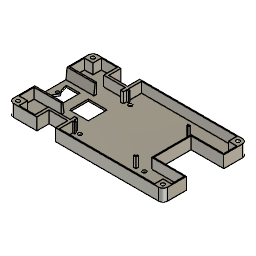
CAR (Autodesk Fusion 360 archive; units mm, degrees)
design "MID"
Autodesk Fusion 360 part; units mm, degrees
(part 1 of 2)
sketch "Sketch1" plane through (0, 0, 0) normal (0, 0, 1) x (1, 0, 0)
  line L0 (0, 0) -> (165, 0)
  line L1 (165, 0) -> (165, 90)
  line L2 (165, 90) -> (0, 90)
  line L3 (0, 90) -> (0, 0)
  dimension "d1" = 165
  dimension "d2" = 90
  constraint horizontal L0
  constraint vertical L1
  constraint horizontal L2
  constraint vertical L3
  constraint coincident L0.start L3.end
  measures "d1" distance of L0.start L0.end
  measures "d2" distance of L0.start L2.end
extrude "Extrude1" add sketch "Sketch1" along normal blind 3
sketch "Sketch4" plane through (0, 0, 3) normal (0, 0, 1) x (-1, 0, 0)
  line L0 (-165, 0) -> (-165, -90)
  line L1 (-165, -90) -> (0, -90)
  line L2 (0, -90) -> (0, 0)
  line L3 (0, 0) -> (-165, 0)
  line L4 (-30, -90) -> (-50, -90)
  line L5 (-50, -90) -> (-50, -77)
  line L6 (-50, -77) -> (-30, -77)
  line L7 (-30, -77) -> (-30, -90)
  line L8 (-30, 0) -> (-50, 0)
  line L9 (-50, 0) -> (-50, -13)
  line L10 (-50, -13) -> (-30, -13)
  line L11 (-30, -13) -> (-30, 0)
  dimension "d9" = 20
  dimension "d10" = 13
  dimension "d11" = 20
  dimension "d12" = 13
  constraint horizontal L4
  constraint vertical L5
  constraint horizontal L6
  constraint vertical L7
  constraint coincident L1 L4.start
  constraint horizontal L8
  constraint vertical L9
  constraint horizontal L10
  constraint vertical L11
  constraint coincident L3 L8.start
  measures "d9" distance of L4.start L4.end
  measures "d10" distance of L4.start L6.end
  measures "d11" distance of L8.start L8.end
  measures "d12" distance of L8.start L10.end
extrude "Extrude2" cut sketch "Sketch4" against normal blind 3 contours L3 L8 L9 L10 L11 | L1 L4 L5 L6 L7
sketch "Sketch6" plane through (0, 0, 3) normal (0, 0, 1) x (-1, 0, 0)
  line L0 (-30, -77) -> (-30, -90)
  line L1 (-30, -90) -> (0, -90)
  line L2 (0, -90) -> (0, 0)
  line L3 (0, 0) -> (-30, 0)
  line L4 (-30, 0) -> (-30, -13)
  line L5 (-30, -13) -> (-50, -13)
  line L6 (-50, -13) -> (-50, 0)
  line L7 (-50, 0) -> (-165, 0)
  line L8 (-165, 0) -> (-165, -90)
  line L9 (-50, -90) -> (-50, -77)
  line L10 (-50, -77) -> (-30, -77)
  line L11 (-5, -45) -> (-5, -60)
  line L12 (-5, -60) -> (-20, -60)
  line L13 (-20, -60) -> (-20, -30)
  line L14 (-20, -30) -> (-5, -30)
  line L15 (-5, -30) -> (-5, -45)
  line L16 (0, -65) -> (-25, -65)
  line L17 (-25, -65) -> (-25, -25)
  line L18 (-25, -25) -> (0, -25)
  line L19 (0, -25) -> (0, -65)
  line L20 (-165, -90) -> (-50, -90)
  dimension "d20" = 15
  dimension "d21" = 15
  constraint parallel L2 L11
  constraint perpendicular L2 L12
  constraint perpendicular L12 L13
  constraint perpendicular L2 L14
  constraint perpendicular L14 L15
  constraint horizontal L16
  constraint vertical L17
  constraint horizontal L18
  constraint vertical L19
  constraint coincident L2 L16.start
  measures "d20" distance of L11.start L11.end
  measures "d21" distance of L11.end L12.end
extrude "Extrude4" add sketch "Sketch6" along normal blind 10 contours L2 L16 L17 L18 L19
sketch "Sketch7" plane through (0, 0, 3) normal (0, 0, 1) x (-1, 0, 0)
  line L0 (0, -65) -> (-25, -65)
  line L1 (-25, -65) -> (-25, -25)
  line L2 (-25, -25) -> (0, -25)
  line L3 (0, -25) -> (0, 0)
  line L4 (0, 0) -> (-30, 0)
  line L5 (-30, 0) -> (-30, -13)
  line L6 (-30, -13) -> (-50, -13)
  line L7 (-50, -13) -> (-50, 0)
  line L8 (-50, 0) -> (-165, 0)
  line L9 (-165, 0) -> (-165, -90)
  line L10 (-165, -90) -> (-50, -90)
  line L11 (-50, -90) -> (-50, -77)
  line L12 (-50, -77) -> (-30, -77)
  line L13 (-30, -77) -> (-30, -90)
  line L14 (-30, -90) -> (0, -90)
  line L15 (-25, 0) -> (-55, 0)
  line L16 (-55, 0) -> (-55, -15)
  line L17 (-55, -15) -> (-25, -15)
  line L18 (-25, -15) -> (-25, 0)
  line L19 (-25, -90) -> (-55, -90)
  line L20 (-55, -90) -> (-55, -75)
  line L21 (-55, -75) -> (-25, -75)
  line L22 (-25, -75) -> (-25, -90)
  line L23 (0, -90) -> (0, -65)
  constraint horizontal L15
  constraint vertical L16
  constraint horizontal L17
  constraint vertical L18
  constraint coincident L4 L15.start
  constraint horizontal L19
  constraint vertical L20
  constraint horizontal L21
  constraint vertical L22
  constraint coincident L14 L19.start
extrude "Extrude5" add sketch "Sketch7" along normal blind 10 contours L10 L11 L12 L13 L14 L19 L20 L21 L22 | L4 L5 L6 L7 L8 L15 L16 L17 L18
sketch "Sketch12" plane through (0, 0, 3) normal (0, 0, 1) x (-1, 0, 0)
  line L0 (-55, -15) -> (-55, 0)
  line L1 (-55, 0) -> (-165, 0)
  line L2 (-165, 0) -> (-165, -90)
  line L3 (-165, -90) -> (-55, -90)
  line L4 (-55, -90) -> (-55, -75)
  line L5 (-55, -75) -> (-25, -75)
  line L6 (-25, -75) -> (-25, -90)
  line L7 (-25, -90) -> (0, -90)
  line L8 (0, -90) -> (0, -65)
  line L9 (0, -65) -> (-25, -65)
  line L10 (-25, -65) -> (-25, -25)
  line L11 (-25, -25) -> (0, -25)
  line L12 (0, -25) -> (0, 0)
  line L13 (0, 0) -> (-25, 0)
  line L14 (-25, 0) -> (-25, -15)
  line L15 (-25, -15) -> (-55, -15)
  line L16 (-25, -90) -> (0, -90)
  line L17 (0, -90) -> (0, -65)
  line L18 (0, -65) -> (-5, -65)
  line L19 (-5, -65) -> (-5, -85)
  line L20 (-5, -85) -> (-25, -85)
  line L21 (-25, -85) -> (-25, -90)
  line L22 (0, -25) -> (0, 0)
  line L23 (0, 0) -> (-25, 0)
  line L24 (-25, 0) -> (-25, -5)
  line L25 (-25, -5) -> (-5, -5)
  line L26 (-5, -5) -> (-5, -25)
  line L27 (-5, -25) -> (0, -25)
  line L28 (-55, -90) -> (-165, -90)
  line L29 (-165, -90) -> (-165, 0)
  line L30 (-165, 0) -> (-55, 0)
  line L31 (-55, 0) -> (-55, -5)
  line L32 (-55, -5) -> (-160, -5)
  line L33 (-160, -5) -> (-160, -85)
  line L34 (-160, -85) -> (-55, -85)
  line L35 (-55, -90) -> (-55, -85)
  constraint coincident L6.end L7.start
  constraint coincident L7.end L8.start
  constraint coincident L8.end L9.start
  constraint coincident L9 L18.end
  constraint perpendicular L18 L19
  constraint coincident L6 L20.end
  constraint perpendicular L6 L20
  constraint coincident L11.end L12.start
  constraint coincident L12.end L13.start
  constraint coincident L13.end L14.start
  constraint coincident L14 L24.end
  constraint perpendicular L24 L25
  constraint coincident L11 L26.end
  constraint perpendicular L11 L26
  constraint coincident L3.end L4.start
  constraint coincident L2.end L3.start
  constraint coincident L1.end L2.start
  constraint coincident L0.end L1.start
  constraint coincident L0 L31.end
  constraint perpendicular L31 L32
  constraint perpendicular L32 L33
  constraint coincident L4 L34.end
  constraint perpendicular L4 L34
extrude "Extrude9" add sketch "Sketch12" along normal blind 10 contours L0 L1 L2 L3 L4 L28 L29 L30 L31 L32 L33 L34 L35 | L11 L12 L13 L14 L22 L23 L24 L25 L26 L27 | L6 L7 L8 L9 L16 L17 L18 L19 L20 L21
fillet "Fillet6" radius 5 4 edges at (0, 0, 6.5) (165, 0, 6.5) (165, 90, 6.5) (0, 90, 6.5)
extrude "Extrude10" add 1 faces at (45, 75, 6.3333) along direction (0, -1, 0) blind 2.5
extrude "Extrude11" add 1 faces at (45, 15, 6.3333) along direction (0, 1, 0) blind 2.5
extrude "Extrude12" cut 1 faces at (10, 40, 3) along direction (0, 0, -1) blind 3
sketch "Sketch13" plane through (0, 0, 3) normal (0, 0, 1) x (-1, 0, 0)
  line L0 (-55, -17.5) -> (-55, -5)
  line L1 (-55, -5) -> (-160, -5)
  line L2 (-160, -5) -> (-160, -85)
  line L3 (-160, -85) -> (-55, -85)
  line L4 (-55, -85) -> (-55, -72.5)
  line L5 (-55, -72.5) -> (-25, -72.5)
  line L6 (-25, -72.5) -> (-25, -85)
  line L7 (-25, -85) -> (-5, -85)
  line L8 (-5, -85) -> (-5, -65)
  line L9 (-5, -65) -> (-25, -65)
  line L10 (-25, -65) -> (-25, -25)
  line L11 (-25, -25) -> (-5, -25)
  line L12 (-5, -25) -> (-5, -5)
  line L13 (-5, -5) -> (-25, -5)
  line L14 (-25, -5) -> (-25, -17.5)
  line L15 (-25, -17.5) -> (-55, -17.5)
  line L16 (-30, -55) -> (-50, -55)
  line L17 (-50, -55) -> (-50, -35)
  line L18 (-50, -35) -> (-30, -35)
  line L19 (-30, -35) -> (-30, -55)
  constraint horizontal L16
  constraint vertical L17
  constraint horizontal L18
  constraint vertical L19
extrude "Extrude13" cut sketch "Sketch13" against normal blind 3 contours L16 L17 L18 L19
sketch "Sketch15" plane through (0, 0, 3) normal (0, 0, 1) x (-1, 0, 0)
  line L0 (-50, -55) -> (-50, -35)
  line L1 (-50, -35) -> (-30, -35)
  line L2 (-30, -35) -> (-30, -55)
  line L3 (-30, -55) -> (-50, -55)
  line L4 (-55, -17.5) -> (-55, -5)
  line L5 (-55, -5) -> (-160, -5)
  line L6 (-160, -5) -> (-160, -85)
  line L7 (-160, -85) -> (-55, -85)
  line L8 (-55, -85) -> (-55, -72.5)
  line L9 (-55, -72.5) -> (-25, -72.5)
  line L10 (-25, -72.5) -> (-25, -85)
  line L11 (-25, -85) -> (-5, -85)
  line L12 (-5, -85) -> (-5, -65)
  line L13 (-5, -65) -> (-25, -65)
  line L14 (-25, -65) -> (-25, -25)
  line L15 (-25, -25) -> (-5, -25)
  line L16 (-5, -25) -> (-5, -5)
  line L17 (-5, -5) -> (-25, -5)
  line L18 (-25, -5) -> (-25, -17.5)
  line L19 (-25, -17.5) -> (-55, -17.5)
  line L20 (-5, -85) -> (-10, -85)
  line L21 (-10, -85) -> (-10, -80)
  line L22 (-10, -80) -> (-5, -80)
  line L23 (-5, -80) -> (-5, -85)
  line L24 (-5, -10) -> (-10, -10)
  line L25 (-10, -10) -> (-10, -5)
  line L26 (-10, -5) -> (-5, -5)
  line L27 (-5, -5) -> (-5, -10)
  line L28 (-155, -85) -> (-160, -85)
  line L29 (-160, -85) -> (-160, -80)
  line L30 (-160, -80) -> (-155, -80)
  line L31 (-155, -80) -> (-155, -85)
  line L32 (-155, -10) -> (-160, -10)
  line L33 (-160, -10) -> (-160, -5)
  line L34 (-160, -5) -> (-155, -5)
  line L35 (-155, -5) -> (-155, -10)
  constraint horizontal L20
  constraint vertical L21
  constraint horizontal L22
  constraint vertical L23
  constraint coincident L11.end L12.start
  constraint horizontal L24
  constraint vertical L25
  constraint horizontal L26
  constraint vertical L27
  constraint coincident L17 L25.end
  constraint coincident L16 L24.start
  constraint horizontal L28
  constraint vertical L29
  constraint horizontal L30
  constraint vertical L31
  constraint coincident L6 L29.end
  constraint coincident L7 L28.start
  constraint horizontal L32
  constraint vertical L33
  constraint horizontal L34
  constraint vertical L35
  constraint coincident L6 L5.end
extrude "Extrude14" add sketch "Sketch15" along normal blind 10 contours L5 L6 L32 L33 L34 L35 | L16 L17 L24 L25 L26 L27 | L6 L7 L28 L29 L30 L31 | L11 L12 L20 L21 L22 L23
sketch "Sketch16" plane through (0, 0, 13) normal (0, 0, 1) x (-1, 0, 0)
  line L0 (-55, -5) -> (-55, -17.5)
  line L1 (-55, -17.5) -> (-25, -17.5)
  line L2 (-25, -17.5) -> (-25, -5)
  line L3 (-25, -5) -> (-10, -5)
  line L4 (-10, -5) -> (-10, -10)
  line L5 (-10, -10) -> (-5, -10)
  line L6 (-5, -10) -> (-5, -25)
  line L7 (-5, -25) -> (-25, -25)
  line L8 (-25, -25) -> (-25, -65)
  line L9 (-25, -65) -> (-5, -65)
  line L10 (-5, -65) -> (-5, -80)
  line L11 (-5, -80) -> (-10, -80)
  line L12 (-10, -80) -> (-10, -85)
  line L13 (-10, -85) -> (-25, -85)
  line L14 (-25, -85) -> (-25, -72.5)
  line L15 (-25, -72.5) -> (-55, -72.5)
  line L16 (-55, -72.5) -> (-55, -85)
  line L17 (-55, -85) -> (-155, -85)
  line L18 (-155, -85) -> (-155, -80)
  line L19 (-155, -80) -> (-160, -80)
  line L20 (-160, -80) -> (-160, -10)
  line L21 (-160, -10) -> (-155, -10)
  line L22 (-155, -10) -> (-155, -5)
  line L23 (-155, -5) -> (-55, -5)
  line L24 (-20, -30) -> (-5, -30)
  line L25 (-5, -30) -> (-5, -60)
  line L26 (-5, -60) -> (-20, -60)
  line L27 (-20, -60) -> (-20, -30)
  arc A0 (-5, -90) -> (0, -85) centre (-5, -85) ccw
  line L28 (0, -85) -> (0, -5)
  arc A1 (0, -5) -> (-5, 0) centre (-5, -5) ccw
  line L29 (-5, 0) -> (-30, 0)
  line L30 (-30, 0) -> (-30, -13)
  line L31 (-30, -13) -> (-50, -13)
  line L32 (-50, -13) -> (-50, 0)
  line L33 (-50, 0) -> (-160, 0)
  arc A2 (-160, 0) -> (-165, -5) centre (-160, -5) ccw
  line L34 (-165, -5) -> (-165, -85)
  arc A3 (-165, -85) -> (-160, -90) centre (-160, -85) ccw
  line L35 (-160, -90) -> (-50, -90)
  line L36 (-50, -90) -> (-50, -77)
  line L37 (-50, -77) -> (-30, -77)
  line L38 (-30, -77) -> (-30, -90)
  line L39 (-30, -90) -> (-5, -90)
  circle A4 centre (-5, -85) radius 2
  circle A5 centre (-5, -5) radius 2
  circle A6 centre (-160, -85) radius 2
  circle A7 centre (-160, -5) radius 2
  dimension "d52" = 4
  dimension "d53" = 4
  dimension "d54" = 4
  dimension "d55" = 4
  constraint concentric A0 A4
  constraint concentric A1 A5
  constraint concentric A3 A6
  constraint concentric A2 A7
  measures "d52" diameter of A4
  measures "d53" diameter of A5
  measures "d54" diameter of A6
  measures "d55" diameter of A7
extrude "Extrude15" cut sketch "Sketch16" against normal blind 13 contours A4 | A5 | A6 | A7
sketch "Sketch17" plane through (0, 0, 3) normal (0, 0, 1) x (-1, 0, 0)
  line L0 (-50, -55) -> (-50, -35)
  line L1 (-50, -35) -> (-30, -35)
  line L2 (-30, -35) -> (-30, -55)
  line L3 (-30, -55) -> (-50, -55)
  line L4 (-160, -80) -> (-155, -80)
  line L5 (-155, -80) -> (-155, -85)
  line L6 (-155, -85) -> (-55, -85)
  line L7 (-55, -85) -> (-55, -72.5)
  line L8 (-55, -72.5) -> (-25, -72.5)
  line L9 (-25, -72.5) -> (-25, -85)
  line L10 (-25, -85) -> (-10, -85)
  line L11 (-10, -85) -> (-10, -80)
  line L12 (-10, -80) -> (-5, -80)
  line L13 (-5, -80) -> (-5, -65)
  line L14 (-5, -65) -> (-25, -65)
  line L15 (-25, -65) -> (-25, -25)
  line L16 (-25, -25) -> (-5, -25)
  line L17 (-5, -25) -> (-5, -10)
  line L18 (-5, -10) -> (-10, -10)
  line L19 (-10, -10) -> (-10, -5)
  line L20 (-10, -5) -> (-25, -5)
  line L21 (-25, -5) -> (-25, -17.5)
  line L22 (-25, -17.5) -> (-55, -17.5)
  line L23 (-55, -17.5) -> (-55, -5)
  line L24 (-55, -5) -> (-155, -5)
  line L25 (-155, -5) -> (-155, -10)
  line L26 (-155, -10) -> (-160, -10)
  line L27 (-160, -10) -> (-160, -80)
  line L28 (-65, -73) -> (-129, -73)
  line L29 (-129, -73) -> (-129, -17)
  line L30 (-129, -17) -> (-65, -17)
  line L31 (-65, -17) -> (-65, -73)
  line L32 (-60, -78) -> (-134, -78)
  line L33 (-134, -78) -> (-134, -12)
  line L34 (-134, -12) -> (-60, -12)
  line L35 (-60, -12) -> (-60, -78)
  dimension "d58" = 64
  dimension "d59" = 56
  dimension "d60" = 74
  dimension "d61" = 66
  constraint horizontal L28
  constraint vertical L29
  constraint horizontal L30
  constraint vertical L31
  constraint horizontal L32
  constraint vertical L33
  constraint horizontal L34
  constraint vertical L35
  measures "d58" distance of L28.start L28.end
  measures "d59" distance of L28.start L30.end
  measures "d60" distance of L32.start L32.end
  measures "d61" distance of L32.start L34.end
extrude "Extrude18" add 1 faces at (10, 30, 8.6667) along direction (0, 1, 0) blind 4
extrude "Extrude19" add 1 faces at (15, 60, 8.6667) along direction (0, -1, 0) blind 4
extrude "Extrude20" cut 1 faces at (18.3333, 25, 6.3333) along direction (0, 1, 0) blind 4
extrude "Extrude21" cut 1 faces at (11.6667, 65, 6.3333) along direction (0, -1, 0) blind 4
sketch "Sketch19" plane through (0, 0, 0) normal (0, 0, 1) x (1, 0, 0)
  spline S0 degree 5 poles (5, 34) (5.1175, 33.9082) (5.3447, 33.8543) (5.6451, 34.1512) (5.923, 35.197) (6.2299, 37.171) (6.6925, 39.3464) (7.4607, 41.3157) (8.4564, 42.8586) (9.4177, 43.9473) (10.0442, 44.686) (10.0986, 45.2722) (9.5576, 45.9525) (8.6258, 46.9693) (7.5898, 48.4821) (6.7224, 50.5039) (6.1493, 52.81) (5.7864, 54.9179) (5.4759, 56.2775) (5.0616, 56.4098) (4.5396, 55.0911) (4.0446, 52.4587) (3.6617, 48.8489) (3.4755, 44.7456) (3.5326, 40.6932) (3.848, 37.226) (4.2676, 35.2762) (4.6394, 34.4052) (4.8825, 34.0918) (5, 34) knots 0 0 0 0 0 0 0.04 0.08 0.12 0.16 0.2 0.24 0.28 0.32 0.36 0.4 0.44 0.48 0.52 0.56 0.6 0.64 0.68 0.72 0.76 0.8 0.84 0.88 0.92 0.96 1 1 1 1 1 1
  line L0 (4.4073, 34.463) -> (5.5927, 33.537)
  line L1 (5.3989, 56.5988) -> (4.6011, 55.4012)
  point P0 (7, 40)
  point P1 (10, 45)
  point P2 (7, 50)
  point P3 (5, 56)
  constraint midpoint S0.start L0
  constraint midpoint P3 L1
extrude "Extrude22" add sketch "Sketch19" along normal blind 3
sketch "Sketch20" plane through (0, 0, 0) normal (0, 0, -1) x (1, 0, 0)
  arc A0 (0, -85) -> (5, -90) centre (5, -85) ccw
  line L0 (5, -90) -> (30, -90)
  line L1 (30, -90) -> (30, -77)
  line L2 (30, -77) -> (50, -77)
  line L3 (50, -77) -> (50, -90)
  line L4 (50, -90) -> (160, -90)
  arc A1 (160, -90) -> (165, -85) centre (160, -85) ccw
  line L5 (165, -85) -> (165, -5)
  arc A2 (165, -5) -> (160, 0) centre (160, -5) ccw
  line L6 (160, 0) -> (50, 0)
  line L7 (50, 0) -> (50, -13)
  line L8 (50, -13) -> (30, -13)
  line L9 (30, -13) -> (30, 0)
  line L10 (30, 0) -> (5, 0)
  arc A3 (5, 0) -> (0, -5) centre (5, -5) ccw
  line L11 (0, -5) -> (0, -85)
  line L12 (50, -35) -> (50, -55)
  line L13 (50, -55) -> (30, -55)
  line L14 (30, -55) -> (30, -35)
  line L15 (30, -35) -> (50, -35)
  circle A4 centre (5, -85) radius 2
  circle A5 centre (160, -85) radius 2
  circle A6 centre (5, -5) radius 2
  circle A7 centre (160, -5) radius 2
  spline S0 degree 5 poles (5.399, -34) (5.4257, -34.0237) (5.5488, -34.1551) (5.7455, -34.5509) (5.9678, -35.4853) (6.2299, -37.171) (6.6925, -39.3464) (7.4607, -41.3157) (8.4564, -42.8586) (9.4177, -43.9473) (10.0442, -44.686) (10.0986, -45.2722) (9.5576, -45.9525) (8.6258, -46.9693) (7.5898, -48.4821) (6.7224, -50.5039) (6.1493, -52.81) (5.8561, -54.5129) (5.6598, -55.4485) (5.5168, -55.8531) (5.4396, -55.9947) (5.4367, -56) knots 0.029213 0.029213 0.029213 0.029213 0.029213 0.029213 0.04 0.08 0.12 0.16 0.2 0.24 0.28 0.32 0.36 0.4 0.44 0.48 0.52 0.56 0.6 0.64 0.641569 0.641569 0.641569 0.641569 0.641569 0.641569
  line L16 (5.399, -34) -> (20, -34)
  line L17 (20, -34) -> (20, -56)
  line L18 (20, -56) -> (5.4367, -56)
  circle A8 centre (7, -45) radius 1.5
  dimension "d76" = 3
  measures "d76" diameter of A8
extrude "Extrude23" cut sketch "Sketch20" against normal blind 3 contours A8
extrude "Extrude26" add 1 faces at (18.3333, 29, 6.3333) along direction (0, -1, 0) blind 4
extrude "Extrude27" add 1 faces at (11.6667, 61, 6.3333) along direction (0, 1, 0) blind 4
sketch "Sketch23" plane through (0, 34, 0) normal (0, 1, 0) x (-1, 0, 0)
  line L0 (-5.399, 3) -> (-5, 3)
  line L1 (-5, 3) -> (-5, 13)
  line L2 (-5, 13) -> (-20, 13)
  line L3 (-20, 13) -> (-20, 0)
  line L4 (-20, 0) -> (-5.399, 0)
  line L5 (-5.399, 0) -> (-5.399, 3)
  line L6 (-20, 13) -> (-5, 13)
  line L7 (-5, 13) -> (-5, 3)
  line L8 (-5, 3) -> (-20, 3)
  line L9 (-20, 3) -> (-20, 13)
  dimension "d97" = 15
  dimension "d98" = 10
  constraint horizontal L6
  constraint vertical L7
  constraint horizontal L8
  constraint vertical L9
  constraint coincident L2.end L3.start
  measures "d97" distance of L2.end L1.end
  measures "d98" distance of L2.end L8.end
extrude "Extrude28" cut sketch "Sketch23" against normal blind 4 contours L0 L1 L2 L3 L6 L7 L8 L9
sketch "Sketch24" plane through (0, 56, 0) normal (0, -1, 0) x (1, 0, 0)
  line L0 (5.4367, 3) -> (5.4367, 0)
  line L1 (5.4367, 0) -> (20, 0)
  line L2 (20, 0) -> (20, 13)
  line L3 (20, 13) -> (5, 13)
  line L4 (5, 13) -> (5, 3)
  line L5 (5, 3) -> (5.4367, 3)
  line L6 (20, 13) -> (5, 13)
  line L7 (5, 13) -> (5, 3)
  line L8 (5, 3) -> (20, 3)
  line L9 (20, 3) -> (20, 13)
  dimension "d101" = 15
  dimension "d102" = 10
  constraint horizontal L6
  constraint vertical L7
  constraint horizontal L8
  constraint vertical L9
  constraint coincident L2.end L3.start
  measures "d101" distance of L2.end L3.end
  measures "d102" distance of L2.end L8.end
extrude "Extrude29" cut sketch "Sketch24" against normal blind 4 contours L2 L3 L4 L5 L6 L7 L8 L9
sketch "Sketch25" plane through (0, 0, 0) normal (0, 0, -1) x (1, 0, 0)
  circle A0 centre (7, -45) radius 1.5
  arc A1 (0, -85) -> (5, -90) centre (5, -85) ccw
  line L0 (5, -90) -> (30, -90)
  line L1 (30, -90) -> (30, -77)
  line L2 (30, -77) -> (50, -77)
  line L3 (50, -77) -> (50, -90)
  line L4 (50, -90) -> (160, -90)
  arc A2 (160, -90) -> (165, -85) centre (160, -85) ccw
  line L5 (165, -85) -> (165, -5)
  arc A3 (165, -5) -> (160, 0) centre (160, -5) ccw
  line L6 (160, 0) -> (50, 0)
  line L7 (50, 0) -> (50, -13)
  line L8 (50, -13) -> (30, -13)
  line L9 (30, -13) -> (30, 0)
  line L10 (30, 0) -> (5, 0)
  arc A4 (5, 0) -> (0, -5) centre (5, -5) ccw
  line L11 (0, -5) -> (0, -85)
  line L12 (50, -35) -> (50, -55)
  line L13 (50, -55) -> (30, -55)
  line L14 (30, -55) -> (30, -35)
  line L15 (30, -35) -> (50, -35)
  circle A5 centre (5, -85) radius 2
  circle A6 centre (160, -85) radius 2
  circle A7 centre (5, -5) radius 2
  circle A8 centre (160, -5) radius 2
  spline S0 degree 5 poles (5.399, -34) (5.4257, -34.0237) (5.5488, -34.1551) (5.7455, -34.5509) (5.9678, -35.4853) (6.2299, -37.171) (6.6925, -39.3464) (7.4607, -41.3157) (8.4564, -42.8586) (9.4177, -43.9473) (10.0442, -44.686) (10.0986, -45.2722) (9.5576, -45.9525) (8.6258, -46.9693) (7.5898, -48.4821) (6.7224, -50.5039) (6.1493, -52.81) (5.8561, -54.5129) (5.6598, -55.4485) (5.5168, -55.8531) (5.4396, -55.9947) (5.4367, -56) knots 0.029213 0.029213 0.029213 0.029213 0.029213 0.029213 0.04 0.08 0.12 0.16 0.2 0.24 0.28 0.32 0.36 0.4 0.44 0.48 0.52 0.56 0.6 0.64 0.641569 0.641569 0.641569 0.641569 0.641569 0.641569
  line L16 (5.399, -34) -> (20, -34)
  line L17 (20, -34) -> (20, -56)
  line L18 (20, -56) -> (5.4367, -56)
  line L19 (30, -90) -> (50, -90)
  line L20 (50, -90) -> (50, -64)
  line L21 (50, -64) -> (30, -64)
  line L22 (30, -64) -> (30, -90)
  line L23 (30, 0) -> (50, 0)
  line L24 (50, 0) -> (50, -26)
  line L25 (50, -26) -> (30, -26)
  line L26 (30, -26) -> (30, 0)
  dimension "d105" = 20
  dimension "d106" = 26
  dimension "d107" = 20
  dimension "d108" = 26
  constraint horizontal L19
  constraint vertical L20
  constraint horizontal L21
  constraint vertical L22
  constraint coincident L0.end L1.start
  constraint horizontal L23
  constraint vertical L24
  constraint horizontal L25
  constraint vertical L26
  constraint coincident L9.end L10.start
  measures "d105" distance of L0.end L3.end
  measures "d106" distance of L0.end L21.end
  measures "d107" distance of L9.end L6.end
  measures "d108" distance of L9.end L25.end
sketch "Sketch27" plane through (0, 0, 3) normal (0, 0, 1) x (-1, 0, 0)
  line L0 (-50, -55) -> (-50, -35)
  line L1 (-50, -35) -> (-30, -35)
  line L2 (-30, -35) -> (-30, -55)
  line L3 (-30, -55) -> (-50, -55)
  line L4 (-5, -65) -> (-25, -65)
  line L5 (-25, -65) -> (-25, -25)
  line L6 (-25, -25) -> (-5, -25)
  line L7 (-5, -25) -> (-5, -10)
  line L8 (-5, -10) -> (-10, -10)
  line L9 (-10, -10) -> (-10, -5)
  line L10 (-10, -5) -> (-25, -5)
  line L11 (-25, -5) -> (-25, -17.5)
  line L12 (-25, -17.5) -> (-55, -17.5)
  line L13 (-55, -17.5) -> (-55, -5)
  line L14 (-55, -5) -> (-155, -5)
  line L15 (-155, -5) -> (-155, -10)
  line L16 (-155, -10) -> (-160, -10)
  line L17 (-160, -10) -> (-160, -80)
  line L18 (-160, -80) -> (-155, -80)
  line L19 (-155, -80) -> (-155, -85)
  line L20 (-155, -85) -> (-55, -85)
  line L21 (-55, -85) -> (-55, -72.5)
  line L22 (-55, -72.5) -> (-25, -72.5)
  line L23 (-25, -72.5) -> (-25, -85)
  line L24 (-25, -85) -> (-10, -85)
  line L25 (-10, -85) -> (-10, -80)
  line L26 (-10, -80) -> (-5, -80)
  line L27 (-5, -80) -> (-5, -65)
  circle A0 centre (-141, -19) radius 3
  circle A1 centre (-141, -71) radius 3
  circle A2 centre (-73, -19) radius 3
  circle A3 centre (-73, -71) radius 3
  dimension "d113" = 6
  dimension "d114" = 6
  measures "d113" diameter of A0
  measures "d114" diameter of A2
extrude "Extrude34" cut 1 faces at (121.6667, 85, 6.3333) along direction (0, 1, 0) blind 4
extrude "Extrude35" cut 1 faces at (160, 33.3333, 6.3333) along direction (1, 0, 0) blind 4
extrude "Extrude36" cut 1 faces at (88.3333, 5, 6.3333) along direction (0, -1, 0) blind 4
extrude "Extrude37" cut 2 faces at (55, 3.6667, 6.3333) (55, 13.3333, 9.6667) along direction (-1, 0, 0) blind 2
extrude "Extrude38" cut 1 faces at (25, 13.3333, 9.6667) along direction (1, 0, 0) blind 2
extrude "Extrude39" cut 1 faces at (44.3333, 17.5, 6.3333) along direction (0, -1, 0) blind 2
extrude "Extrude40" cut 1 faces at (25, 76.6667, 6.3333) along direction (1, 0, 0) blind 2
extrude "Extrude41" cut 1 faces at (55, 78, 9.6667) along direction (-1, 0, 0) blind 2
extrude "Extrude42" cut 1 faces at (44.3333, 72.5, 6.3333) along direction (0, 1, 0) blind 2
extrude "Extrude43" cut 1 faces at (15.6667, 85, 6.3333) along direction (0, 1, 0) blind 4
extrude "Extrude44" cut 1 faces at (5, 70, 6.3333) along direction (-1, 0, 0) blind 4
extrude "Extrude45" cut 1 faces at (5, 15, 6.3333) along direction (-1, 0, 0) blind 4
extrude "Extrude46" cut 1 faces at (21.3333, 5, 9.6667) along direction (0, -1, 0) blind 4
sketch "Sketch28" plane through (0, 0, 13) normal (0, 0, 1) x (-1, 0, 0)
  line L0 (-10, -1) -> (-10, -10)
  line L1 (-10, -10) -> (-1, -10)
  line L2 (-1, -10) -> (-1, -25)
  line L3 (-1, -25) -> (-25, -25)
  line L4 (-25, -25) -> (-25, -65)
  line L5 (-25, -65) -> (-1, -65)
  line L6 (-1, -65) -> (-1, -80)
  line L7 (-1, -80) -> (-10, -80)
  line L8 (-10, -80) -> (-10, -89)
  line L9 (-10, -89) -> (-27, -89)
  line L10 (-27, -89) -> (-27, -74.5)
  line L11 (-27, -74.5) -> (-53, -74.5)
  line L12 (-53, -74.5) -> (-53, -89)
  line L13 (-53, -89) -> (-155, -89)
  line L14 (-155, -89) -> (-155, -80)
  line L15 (-155, -80) -> (-164, -80)
  line L16 (-164, -80) -> (-164, -10)
  line L17 (-164, -10) -> (-155, -10)
  line L18 (-155, -10) -> (-155, -1)
  line L19 (-155, -1) -> (-53, -1)
  line L20 (-53, -1) -> (-53, -15.5)
  line L21 (-53, -15.5) -> (-27, -15.5)
  line L22 (-27, -15.5) -> (-27, -1)
  line L23 (-27, -1) -> (-10, -1)
  circle A0 centre (-160, -5) radius 2
  circle A1 centre (-5, -5) radius 2
  circle A2 centre (-160, -85) radius 2
  circle A3 centre (-5, -85) radius 2
  line L24 (-5, -30) -> (-5, -60)
  line L25 (-5, -60) -> (-20, -60)
  line L26 (-20, -60) -> (-20, -30)
  line L27 (-20, -30) -> (-5, -30)
  arc A4 (-5, -90) -> (0, -85) centre (-5, -85) ccw
  line L28 (0, -85) -> (0, -5)
  arc A5 (0, -5) -> (-5, 0) centre (-5, -5) ccw
  line L29 (-5, 0) -> (-30, 0)
  line L30 (-30, 0) -> (-30, -13)
  line L31 (-30, -13) -> (-50, -13)
  line L32 (-50, -13) -> (-50, 0)
  line L33 (-50, 0) -> (-160, 0)
  arc A6 (-160, 0) -> (-165, -5) centre (-160, -5) ccw
  line L34 (-165, -5) -> (-165, -85)
  arc A7 (-165, -85) -> (-160, -90) centre (-160, -85) ccw
  line L35 (-160, -90) -> (-50, -90)
  line L36 (-50, -90) -> (-50, -77)
  line L37 (-50, -77) -> (-30, -77)
  line L38 (-30, -77) -> (-30, -90)
  line L39 (-30, -90) -> (-5, -90)
  line L40 (-25, -25) -> (-1, -25)
  line L41 (-1, -25) -> (-1, -65)
  line L42 (-1, -65) -> (-25, -65)
  line L43 (-25, -65) -> (-25, -25)
  constraint horizontal L40
  constraint vertical L41
  constraint horizontal L42
  constraint vertical L43
  constraint coincident L5.end L6.start
  constraint coincident L3.end L4.start
extrude "Extrude47" cut sketch "Sketch28" against normal blind 10 contours L3 L4 L5 L40 L41 L42 L43
sketch "Sketch29" plane through (0, 15.5, 0) normal (0, 1, 0) x (-1, 0, 0)
  line L0 (-27, 3) -> (-27, 13)
  line L1 (-27, 13) -> (-53, 13)
  line L2 (-53, 13) -> (-53, 3)
  line L3 (-53, 3) -> (-27, 3)
  line L4 (-53, 13) -> (-50, 13)
  line L5 (-50, 13) -> (-50, 3)
  line L6 (-50, 3) -> (-53, 3)
  line L7 (-53, 3) -> (-53, 13)
  dimension "d147" = 3
  dimension "d148" = 10
  constraint horizontal L4
  constraint vertical L5
  constraint horizontal L6
  constraint vertical L7
  constraint coincident L1.end L2.start
  measures "d147" distance of L1.end L4.end
  measures "d148" distance of L1.end L2.end
extrude "Extrude48" add sketch "Sketch29" along normal blind 5 contours L1 L2 L3 L4 L5 L6 L7
sketch "Sketch30" plane through (0, 74.5, 0) normal (0, -1, 0) x (1, 0, 0)
  line L0 (53, 3) -> (53, 13)
  line L1 (53, 13) -> (27, 13)
  line L2 (27, 13) -> (27, 3)
  line L3 (27, 3) -> (53, 3)
  line L4 (50, 13) -> (53, 13)
  line L5 (53, 13) -> (53, 3)
  line L6 (53, 3) -> (50, 3)
  line L7 (50, 3) -> (50, 13)
  constraint horizontal L4
  constraint vertical L5
  constraint horizontal L6
  constraint vertical L7
  constraint coincident L0.start L3.end
  constraint coincident L1 L4.start
extrude "Extrude49" add sketch "Sketch30" along normal blind 5 contours L0 L1 L3 L4 L5 L6 L7
sketch "Sketch31" plane through (0, 0, 3) normal (0, 0, 1) x (-1, 0, 0)
  line L0 (-50, -69.5) -> (-50, -74.5)
  line L1 (-50, -74.5) -> (-27, -74.5)
  line L2 (-27, -74.5) -> (-27, -89)
  line L3 (-27, -89) -> (-10, -89)
  line L4 (-10, -89) -> (-10, -80)
  line L5 (-10, -80) -> (-1, -80)
  line L6 (-1, -80) -> (-1, -10)
  line L7 (-1, -10) -> (-10, -10)
  line L8 (-10, -10) -> (-10, -1)
  line L9 (-10, -1) -> (-27, -1)
  line L10 (-27, -1) -> (-27, -15.5)
  line L11 (-27, -15.5) -> (-50, -15.5)
  line L12 (-50, -15.5) -> (-50, -20.5)
  line L13 (-50, -20.5) -> (-53, -20.5)
  line L14 (-53, -20.5) -> (-53, -1)
  line L15 (-53, -1) -> (-155, -1)
  line L16 (-155, -1) -> (-155, -10)
  line L17 (-155, -10) -> (-164, -10)
  line L18 (-164, -10) -> (-164, -80)
  line L19 (-164, -80) -> (-155, -80)
  line L20 (-155, -80) -> (-155, -89)
  line L21 (-155, -89) -> (-53, -89)
  line L22 (-53, -89) -> (-53, -69.5)
  line L23 (-53, -69.5) -> (-50, -69.5)
  line L24 (-20, -56) -> (-20, -34)
  line L25 (-20, -34) -> (-5.399, -34)
  spline S0 degree 5 poles (-5.399, -34) (-5.4257, -34.0237) (-5.5488, -34.1551) (-5.7455, -34.5509) (-5.9678, -35.4853) (-6.2299, -37.171) (-6.6925, -39.3464) (-7.4607, -41.3157) (-8.4564, -42.8586) (-9.4177, -43.9473) (-10.0442, -44.686) (-10.0986, -45.2722) (-9.5576, -45.9525) (-8.6258, -46.9693) (-7.5898, -48.4821) (-6.7224, -50.5039) (-6.1493, -52.81) (-5.8561, -54.5129) (-5.6598, -55.4485) (-5.5168, -55.8531) (-5.4396, -55.9947) (-5.4367, -56) knots 0.029213 0.029213 0.029213 0.029213 0.029213 0.029213 0.04 0.08 0.12 0.16 0.2 0.24 0.28 0.32 0.36 0.4 0.44 0.48 0.52 0.56 0.6 0.64 0.641569 0.641569 0.641569 0.641569 0.641569 0.641569
  line L26 (-5.4367, -56) -> (-20, -56)
  circle A0 centre (-7, -45) radius 1.5
  line L27 (-50, -55) -> (-50, -35)
  line L28 (-50, -35) -> (-30, -35)
  line L29 (-30, -35) -> (-30, -55)
  line L30 (-30, -55) -> (-50, -55)
  line L31 (-53, -17) -> (-119, -17)
  line L32 (-119, -17) -> (-119, -73)
  line L33 (-119, -73) -> (-53, -73)
  line L34 (-53, -73) -> (-53, -17)
  line L35 (-117.5, -73) -> (-117.5, -74)
  line L36 (-117.5, -74) -> (-120, -74)
  line L37 (-120, -74) -> (-120, -71.5)
  line L38 (-120, -71.5) -> (-119, -71.5)
  line L39 (-119, -18.5) -> (-120, -18.5)
  line L40 (-120, -18.5) -> (-120, -16)
  line L41 (-120, -16) -> (-117.5, -16)
  line L42 (-117.5, -16) -> (-117.5, -17)
  line L43 (-53, -15.5) -> (-55, -15.5)
  line L44 (-55, -15.5) -> (-55, -17)
  line L45 (-55, -17) -> (-53, -17)
  line L46 (-53, -17) -> (-53, -15.5)
  line L47 (-53, -74.5) -> (-55, -74.5)
  line L48 (-55, -74.5) -> (-55, -73)
  line L49 (-55, -73) -> (-53, -73)
  line L50 (-53, -73) -> (-53, -74.5)
  dimension "d153" = 66
  dimension "d154" = 56
  constraint horizontal L31
  constraint vertical L32
  constraint horizontal L33
  constraint vertical L34
  constraint coincident L14 L31.start
  constraint coincident L33 L35.start
  constraint perpendicular L33 L35
  constraint perpendicular L32 L36
  constraint perpendicular L33 L37
  constraint coincident L32 L38.end
  constraint perpendicular L32 L38
  constraint coincident L32 L39.start
  constraint perpendicular L32 L39
  constraint perpendicular L33 L40
  constraint perpendicular L32 L41
  constraint coincident L31 L42.end
  constraint perpendicular L31 L42
  constraint horizontal L43
  constraint vertical L44
  constraint horizontal L45
  constraint vertical L46
  constraint coincident L31 L44.end
  constraint coincident L14 L43.start
  constraint horizontal L47
  constraint vertical L48
  constraint horizontal L49
  constraint vertical L50
  constraint coincident L33 L48.end
  constraint coincident L22 L47.start
  measures "d153" distance of L31.start L31.end
  measures "d154" distance of L31.start L33.end
extrude "Extrude50" add sketch "Sketch31" along normal blind 10 contours L22 L33 L47 L48 L49 L50 | L14 L31 L43 L44 L45 L46 | L32 L33 L35 L36 L37 L38 | L31 L32 L39 L40 L41 L42
extrude "Extrude51" cut 7 faces at (95, 48.3333, 3) (15.6667, 3.6667, 3) (3.6667, 15, 3) (23.3333, 48.6667, 3) (3.6667, 70, 3) (21.3333, 86.3333, 3) (10.1456, 58.6667, 3) along direction (0, 0, -1) blind 1
sketch "Sketch32" plane through (0, 0, 0) normal (0, 0, -1) x (1, 0, 0)
  circle A0 centre (7, -45) radius 1.5
  arc A1 (0, -85) -> (5, -90) centre (5, -85) ccw
  line L0 (5, -90) -> (30, -90)
  line L1 (30, -90) -> (30, -77)
  line L2 (30, -77) -> (50, -77)
  line L3 (50, -77) -> (50, -90)
  line L4 (50, -90) -> (160, -90)
  arc A2 (160, -90) -> (165, -85) centre (160, -85) ccw
  line L5 (165, -85) -> (165, -5)
  arc A3 (165, -5) -> (160, 0) centre (160, -5) ccw
  line L6 (160, 0) -> (50, 0)
  line L7 (50, 0) -> (50, -13)
  line L8 (50, -13) -> (30, -13)
  line L9 (30, -13) -> (30, 0)
  line L10 (30, 0) -> (5, 0)
  arc A4 (5, 0) -> (0, -5) centre (5, -5) ccw
  line L11 (0, -5) -> (0, -85)
  line L12 (50, -35) -> (50, -55)
  line L13 (50, -55) -> (30, -55)
  line L14 (30, -55) -> (30, -35)
  line L15 (30, -35) -> (50, -35)
  circle A5 centre (5, -85) radius 2
  circle A6 centre (160, -85) radius 2
  circle A7 centre (5, -5) radius 2
  circle A8 centre (160, -5) radius 2
  spline S0 degree 5 poles (5.399, -34) (5.4257, -34.0237) (5.5488, -34.1551) (5.7455, -34.5509) (5.9678, -35.4853) (6.2299, -37.171) (6.6925, -39.3464) (7.4607, -41.3157) (8.4564, -42.8586) (9.4177, -43.9473) (10.0442, -44.686) (10.0986, -45.2722) (9.5576, -45.9525) (8.6258, -46.9693) (7.5898, -48.4821) (6.7224, -50.5039) (6.1493, -52.81) (5.8561, -54.5129) (5.6598, -55.4485) (5.5168, -55.8531) (5.4396, -55.9947) (5.4367, -56) knots 0.029213 0.029213 0.029213 0.029213 0.029213 0.029213 0.04 0.08 0.12 0.16 0.2 0.24 0.28 0.32 0.36 0.4 0.44 0.48 0.52 0.56 0.6 0.64 0.641569 0.641569 0.641569 0.641569 0.641569 0.641569
  line L16 (5.399, -34) -> (20, -34)
  line L17 (20, -34) -> (20, -56)
  line L18 (20, -56) -> (5.4367, -56)
  line L19 (55, -75) -> (130, -75)
  line L20 (130, -75) -> (130, -15)
  line L21 (130, -15) -> (55, -15)
  line L22 (55, -15) -> (55, -75)
  circle A9 centre (127, -18) radius 2
  circle A10 centre (127, -72) radius 2
  circle A11 centre (58, -72) radius 2
  circle A12 centre (58, -18) radius 2
  dimension "d159" = 75
  dimension "d160" = 60
  dimension "d161" = 4
  dimension "d162" = 4
  dimension "d163" = 4
  dimension "d164" = 4
  constraint horizontal L19
  constraint vertical L20
  constraint horizontal L21
  constraint vertical L22
  measures "d159" distance of L19.start L19.end
  measures "d160" distance of L19.start L21.end
  measures "d161" diameter of A9
  measures "d162" diameter of A10
  measures "d163" diameter of A11
  measures "d164" diameter of A12
extrude "Extrude52" cut sketch "Sketch32" against normal blind 3 contours A9 | A10 | A11 | A12
sketch "Sketch33" plane through (0, 0, 13) normal (0, 0, 1) x (-1, 0, 0)
  line L0 (-1, -10) -> (-1, -80)
  line L1 (-1, -80) -> (-10, -80)
  line L2 (-10, -80) -> (-10, -89)
  line L3 (-10, -89) -> (-27, -89)
  line L4 (-27, -89) -> (-27, -74.5)
  line L5 (-27, -74.5) -> (-50, -74.5)
  line L6 (-50, -74.5) -> (-50, -69.5)
  line L7 (-50, -69.5) -> (-53, -69.5)
  line L8 (-53, -69.5) -> (-53, -73)
  line L9 (-53, -73) -> (-55, -73)
  line L10 (-55, -73) -> (-55, -74.5)
  line L11 (-55, -74.5) -> (-53, -74.5)
  line L12 (-53, -74.5) -> (-53, -89)
  line L13 (-53, -89) -> (-155, -89)
  line L14 (-155, -89) -> (-155, -80)
  line L15 (-155, -80) -> (-164, -80)
  line L16 (-164, -80) -> (-164, -10)
  line L17 (-164, -10) -> (-155, -10)
  line L18 (-155, -10) -> (-155, -1)
  line L19 (-155, -1) -> (-53, -1)
  line L20 (-53, -1) -> (-53, -15.5)
  line L21 (-53, -15.5) -> (-55, -15.5)
  line L22 (-55, -15.5) -> (-55, -17)
  line L23 (-55, -17) -> (-53, -17)
  line L24 (-53, -17) -> (-53, -20.5)
  line L25 (-53, -20.5) -> (-50, -20.5)
  line L26 (-50, -20.5) -> (-50, -15.5)
  line L27 (-50, -15.5) -> (-27, -15.5)
  line L28 (-27, -15.5) -> (-27, -1)
  line L29 (-27, -1) -> (-10, -1)
  line L30 (-10, -1) -> (-10, -10)
  line L31 (-10, -10) -> (-1, -10)
  circle A0 centre (-160, -5) radius 2
  circle A1 centre (-5, -5) radius 2
  circle A2 centre (-160, -85) radius 2
  circle A3 centre (-5, -85) radius 2
  arc A4 (-5, -90) -> (0, -85) centre (-5, -85) ccw
  line L32 (0, -85) -> (0, -5)
  arc A5 (0, -5) -> (-5, 0) centre (-5, -5) ccw
  line L33 (-5, 0) -> (-30, 0)
  line L34 (-30, 0) -> (-30, -13)
  line L35 (-30, -13) -> (-50, -13)
  line L36 (-50, -13) -> (-50, 0)
  line L37 (-50, 0) -> (-160, 0)
  arc A6 (-160, 0) -> (-165, -5) centre (-160, -5) ccw
  line L38 (-165, -5) -> (-165, -85)
  arc A7 (-165, -85) -> (-160, -90) centre (-160, -85) ccw
  line L39 (-160, -90) -> (-50, -90)
  line L40 (-50, -90) -> (-50, -77)
  line L41 (-50, -77) -> (-30, -77)
  line L42 (-30, -77) -> (-30, -90)
  line L43 (-30, -90) -> (-5, -90)
  line L44 (0, -26) -> (-1, -26)
  line L45 (-1, -26) -> (-1, -64)
  line L46 (-1, -64) -> (0, -64)
  line L47 (0, -64) -> (0, -26)
  dimension "d167" = 1
  dimension "d168" = 38
  constraint horizontal L44
  constraint vertical L45
  constraint horizontal L46
  constraint vertical L47
  constraint coincident L32 L44.start
  measures "d167" distance of L44.start L44.end
  measures "d168" distance of L44.start L46.end
extrude "Extrude53" cut sketch "Sketch33" against normal blind 11 contours L0 L32 L44 L45 L46 L47
sketch "Sketch34" plane through (0, 0, 0) normal (0, 0, -1) x (1, 0, 0)
  circle A0 centre (58, -72) radius 2
  circle A1 centre (58, -18) radius 2
  circle A2 centre (127, -72) radius 2
  circle A3 centre (127, -18) radius 2
  circle A4 centre (7, -45) radius 1.5
  arc A5 (0, -85) -> (5, -90) centre (5, -85) ccw
  line L0 (5, -90) -> (30, -90)
  line L1 (30, -90) -> (30, -77)
  line L2 (30, -77) -> (50, -77)
  line L3 (50, -77) -> (50, -90)
  line L4 (50, -90) -> (160, -90)
  arc A6 (160, -90) -> (165, -85) centre (160, -85) ccw
  line L5 (165, -85) -> (165, -5)
  arc A7 (165, -5) -> (160, 0) centre (160, -5) ccw
  line L6 (160, 0) -> (50, 0)
  line L7 (50, 0) -> (50, -13)
  line L8 (50, -13) -> (30, -13)
  line L9 (30, -13) -> (30, 0)
  line L10 (30, 0) -> (5, 0)
  arc A8 (5, 0) -> (0, -5) centre (5, -5) ccw
  line L11 (0, -5) -> (0, -85)
  line L12 (50, -35) -> (50, -55)
  line L13 (50, -55) -> (30, -55)
  line L14 (30, -55) -> (30, -35)
  line L15 (30, -35) -> (50, -35)
  circle A9 centre (5, -85) radius 2
  circle A10 centre (160, -85) radius 2
  circle A11 centre (5, -5) radius 2
  circle A12 centre (160, -5) radius 2
  spline S0 degree 5 poles (5.399, -34) (5.4257, -34.0237) (5.5488, -34.1551) (5.7455, -34.5509) (5.9678, -35.4853) (6.2299, -37.171) (6.6925, -39.3464) (7.4607, -41.3157) (8.4564, -42.8586) (9.4177, -43.9473) (10.0442, -44.686) (10.0986, -45.2722) (9.5576, -45.9525) (8.6258, -46.9693) (7.5898, -48.4821) (6.7224, -50.5039) (6.1493, -52.81) (5.8561, -54.5129) (5.6598, -55.4485) (5.5168, -55.8531) (5.4396, -55.9947) (5.4367, -56) knots 0.029213 0.029213 0.029213 0.029213 0.029213 0.029213 0.04 0.08 0.12 0.16 0.2 0.24 0.28 0.32 0.36 0.4 0.44 0.48 0.52 0.56 0.6 0.64 0.641569 0.641569 0.641569 0.641569 0.641569 0.641569
  line L16 (5.399, -34) -> (20, -34)
  line L17 (20, -34) -> (20, -56)
  line L18 (20, -56) -> (5.4367, -56)
  line L19 (130, -65) -> (165, -65)
  line L20 (165, -65) -> (165, -25)
  line L21 (165, -25) -> (130, -25)
  line L22 (130, -25) -> (130, -65)
  dimension "d171" = 40
  constraint horizontal L19
  constraint vertical L20
  constraint horizontal L21
  constraint vertical L22
  constraint coincident L5 L20.end
  measures "d171" distance of L19.start L21.end
extrude "Extrude54" cut sketch "Sketch34" against normal blind 13 contours L5 L19 L20 L21 L22
sketch "Sketch35" plane through (0, 0, 2) normal (0, 0, 1) x (-1, 0, 0)
  line L0 (-130, -65) -> (-164, -65)
  line L1 (-164, -65) -> (-164, -80)
  line L2 (-164, -80) -> (-155, -80)
  line L3 (-155, -80) -> (-155, -89)
  line L4 (-155, -89) -> (-53, -89)
  line L5 (-53, -89) -> (-53, -74.5)
  line L6 (-53, -74.5) -> (-55, -74.5)
  line L7 (-55, -74.5) -> (-55, -73)
  line L8 (-55, -73) -> (-53, -73)
  line L9 (-53, -73) -> (-53, -69.5)
  line L10 (-53, -69.5) -> (-50, -69.5)
  line L11 (-50, -69.5) -> (-50, -74.5)
  line L12 (-50, -74.5) -> (-27, -74.5)
  line L13 (-27, -74.5) -> (-27, -89)
  line L14 (-27, -89) -> (-10, -89)
  line L15 (-10, -89) -> (-10, -80)
  line L16 (-10, -80) -> (-1, -80)
  line L17 (-1, -80) -> (-1, -64)
  line L18 (-1, -64) -> (0, -64)
  line L19 (0, -64) -> (0, -26)
  line L20 (0, -26) -> (-1, -26)
  line L21 (-1, -26) -> (-1, -10)
  line L22 (-1, -10) -> (-10, -10)
  line L23 (-10, -10) -> (-10, -1)
  line L24 (-10, -1) -> (-27, -1)
  line L25 (-27, -1) -> (-27, -15.5)
  line L26 (-27, -15.5) -> (-50, -15.5)
  line L27 (-50, -15.5) -> (-50, -20.5)
  line L28 (-50, -20.5) -> (-53, -20.5)
  line L29 (-53, -20.5) -> (-53, -17)
  line L30 (-53, -17) -> (-55, -17)
  line L31 (-55, -17) -> (-55, -15.5)
  line L32 (-55, -15.5) -> (-53, -15.5)
  line L33 (-53, -15.5) -> (-53, -1)
  line L34 (-53, -1) -> (-155, -1)
  line L35 (-155, -1) -> (-155, -10)
  line L36 (-155, -10) -> (-164, -10)
  line L37 (-164, -10) -> (-164, -25)
  line L38 (-164, -25) -> (-130, -25)
  line L39 (-130, -25) -> (-130, -65)
  circle A0 centre (-58, -72) radius 2
  circle A1 centre (-58, -18) radius 2
  circle A2 centre (-127, -72) radius 2
  circle A3 centre (-127, -18) radius 2
  line L40 (-50, -55) -> (-50, -35)
  line L41 (-50, -35) -> (-30, -35)
  line L42 (-30, -35) -> (-30, -55)
  line L43 (-30, -55) -> (-50, -55)
  circle A4 centre (-7, -45) radius 1.5
  line L44 (-20, -56) -> (-20, -34)
  line L45 (-20, -34) -> (-5.399, -34)
  spline S0 degree 3 poles (-5.4367, -56) (-5.7497, -55.4367) (-5.943, -53.6627) (-6.9547, -49.8003) (-7.6102, -48.4226) (-9.0239, -46.5206) (-9.456, -46.0718) (-9.8225, -45.5633) (-9.8989, -45.4352) (-9.9798, -45.2216) (-10.0001, -45.1304) (-10.0013, -44.9324) (-9.9796, -44.8313) (-9.7164, -44.175) (-8.9388, -43.522) (-6.9509, -40.4805) (-6.5375, -38.6632) (-6.0275, -35.9464) (-5.8982, -35.1719) (-5.6737, -34.4616) (-5.6073, -34.2904) (-5.4915, -34.1018) (-5.449, -34.0444) (-5.399, -34) knots -1.464984 -1.464984 -1.464984 -1.464984 -1.220656 -1.220656 -0.966027 -0.966027 -0.834398 -0.834398 -0.784062 -0.784062 -0.747922 -0.747922 -0.709301 -0.709301 -0.507654 -0.507654 -0.20805 -0.20805 -0.066515 -0.066515 -0.020055 -0.020055 0 0 0 0
  line L46 (-5.4367, -56) -> (-20, -56)
  line L47 (-120, -71.5) -> (-119, -71.5)
  line L48 (-119, -71.5) -> (-119, -73)
  line L49 (-119, -73) -> (-117.5, -73)
  line L50 (-117.5, -73) -> (-117.5, -74)
  line L51 (-117.5, -74) -> (-120, -74)
  line L52 (-120, -74) -> (-120, -71.5)
  line L53 (-117.5, -16) -> (-117.5, -17)
  line L54 (-117.5, -17) -> (-119, -17)
  line L55 (-119, -17) -> (-119, -18.5)
  line L56 (-119, -18.5) -> (-120, -18.5)
  line L57 (-120, -18.5) -> (-120, -16)
  line L58 (-120, -16) -> (-117.5, -16)
  line L59 (-164, -24) -> (-129, -24)
  line L60 (-129, -24) -> (-129, -66)
  line L61 (-129, -66) -> (-164, -66)
  line L62 (-164, -66) -> (-164, -24)
  constraint horizontal L59
  constraint vertical L60
  constraint horizontal L61
  constraint vertical L62
  constraint coincident L37 L59.start
extrude "Extrude55" add sketch "Sketch35" along normal blind 11 contours L0 L1 L37 L38 L39 L59 L60 L61 L62
sketch "Sketch36" plane through (0, 0, 2) normal (0, 0, 1) x (-1, 0, 0)
  line L0 (-117.5, -16) -> (-117.5, -17)
  line L1 (-117.5, -17) -> (-119, -17)
  line L2 (-119, -17) -> (-119, -18.5)
  line L3 (-119, -18.5) -> (-120, -18.5)
  line L4 (-120, -18.5) -> (-120, -16)
  line L5 (-120, -16) -> (-117.5, -16)
  line L6 (-120, -71.5) -> (-119, -71.5)
  line L7 (-119, -71.5) -> (-119, -73)
  line L8 (-119, -73) -> (-117.5, -73)
  line L9 (-117.5, -73) -> (-117.5, -74)
  line L10 (-117.5, -74) -> (-120, -74)
  line L11 (-120, -74) -> (-120, -71.5)
  line L12 (-20, -56) -> (-20, -34)
  line L13 (-20, -34) -> (-5.399, -34)
  spline S0 degree 3 poles (-5.4367, -56) (-5.7497, -55.4367) (-5.943, -53.6627) (-6.9547, -49.8003) (-7.6102, -48.4226) (-9.0239, -46.5206) (-9.456, -46.0718) (-9.8225, -45.5633) (-9.8989, -45.4352) (-9.9798, -45.2216) (-10.0001, -45.1304) (-10.0013, -44.9324) (-9.9796, -44.8313) (-9.7164, -44.175) (-8.9388, -43.522) (-6.9509, -40.4805) (-6.5375, -38.6632) (-6.0275, -35.9464) (-5.8982, -35.1719) (-5.6737, -34.4616) (-5.6073, -34.2904) (-5.4915, -34.1018) (-5.449, -34.0444) (-5.399, -34) knots -1.464984 -1.464984 -1.464984 -1.464984 -1.220656 -1.220656 -0.966027 -0.966027 -0.834398 -0.834398 -0.784062 -0.784062 -0.747922 -0.747922 -0.709301 -0.709301 -0.507654 -0.507654 -0.20805 -0.20805 -0.066515 -0.066515 -0.020055 -0.020055 0 0 0 0
  line L14 (-5.4367, -56) -> (-20, -56)
  circle A0 centre (-7, -45) radius 1.5
  line L15 (-50, -55) -> (-50, -35)
  line L16 (-50, -35) -> (-30, -35)
  line L17 (-30, -35) -> (-30, -55)
  line L18 (-30, -55) -> (-50, -55)
  circle A1 centre (-127, -18) radius 2
  circle A2 centre (-127, -72) radius 2
  circle A3 centre (-58, -18) radius 2
  circle A4 centre (-58, -72) radius 2
  line L19 (-164, -24) -> (-129, -24)
  line L20 (-129, -24) -> (-129, -66)
  line L21 (-129, -66) -> (-164, -66)
  line L22 (-164, -66) -> (-164, -80)
  line L23 (-164, -80) -> (-155, -80)
  line L24 (-155, -80) -> (-155, -89)
  line L25 (-155, -89) -> (-53, -89)
  line L26 (-53, -89) -> (-53, -74.5)
  line L27 (-53, -74.5) -> (-55, -74.5)
  line L28 (-55, -74.5) -> (-55, -73)
  line L29 (-55, -73) -> (-53, -73)
  line L30 (-53, -73) -> (-53, -69.5)
  line L31 (-53, -69.5) -> (-50, -69.5)
  line L32 (-50, -69.5) -> (-50, -74.5)
  line L33 (-50, -74.5) -> (-27, -74.5)
  line L34 (-27, -74.5) -> (-27, -89)
  line L35 (-27, -89) -> (-10, -89)
  line L36 (-10, -89) -> (-10, -80)
  line L37 (-10, -80) -> (-1, -80)
  line L38 (-1, -80) -> (-1, -64)
  line L39 (-1, -64) -> (0, -64)
  line L40 (0, -64) -> (0, -26)
  line L41 (0, -26) -> (-1, -26)
  line L42 (-1, -26) -> (-1, -10)
  line L43 (-1, -10) -> (-10, -10)
  line L44 (-10, -10) -> (-10, -1)
  line L45 (-10, -1) -> (-27, -1)
  line L46 (-27, -1) -> (-27, -15.5)
  line L47 (-27, -15.5) -> (-50, -15.5)
  line L48 (-50, -15.5) -> (-50, -20.5)
  line L49 (-50, -20.5) -> (-53, -20.5)
  line L50 (-53, -20.5) -> (-53, -17)
  line L51 (-53, -17) -> (-55, -17)
  line L52 (-55, -17) -> (-55, -15.5)
  line L53 (-55, -15.5) -> (-53, -15.5)
  line L54 (-53, -15.5) -> (-53, -1)
  line L55 (-53, -1) -> (-155, -1)
  line L56 (-155, -1) -> (-155, -10)
  line L57 (-155, -10) -> (-164, -10)
  line L58 (-164, -10) -> (-164, -24)
  line L59 (0, -64) -> (-30, -64)
  line L60 (-30, -64) -> (-30, -26)
  line L61 (-30, -26) -> (0, -26)
  line L62 (0, -26) -> (0, -64)
  dimension "d176" = 30
  dimension "d177" = 38
  constraint horizontal L59
  constraint vertical L60
  constraint horizontal L61
  constraint vertical L62
  constraint coincident L39.end L40.start
  measures "d176" distance of L39.end L59.end
  measures "d177" distance of L39.end L40.end
extrude "Extrude56" add sketch "Sketch36" along normal blind 25 contours L17 L39 L40 L41 L59 L60 L61 L62
sketch "Sketch37" plane through (0, 0, 0) normal (-1, 0, 0) x (0, -1, 0)
  line L0 (-64, 13) -> (-85, 13)
  line L1 (-85, 13) -> (-85, 0)
  line L2 (-85, 0) -> (-5, 0)
  line L3 (-5, 0) -> (-5, 13)
  line L4 (-5, 13) -> (-26, 13)
  line L5 (-26, 13) -> (-26, 27)
  line L6 (-26, 27) -> (-64, 27)
  line L7 (-64, 27) -> (-64, 13)
  line L8 (-61, 2) -> (-29, 2)
  line L9 (-29, 2) -> (-26, 27)
  line L10 (-26, 27) -> (-64, 27)
  line L11 (-64, 27) -> (-61, 2)
  constraint parallel L2 L8
  constraint coincident L5.end L6.start
  constraint coincident L6.end L7.start
extrude "Extrude57" cut sketch "Sketch37" against normal blind 30 contours L6 L8 L9 L10 L11
sketch "Sketch38" plane through (0, 0, 0) normal (-1, 0, 0) x (0, -1, 0)
  line L0 (-26, 27) -> (-29, 2)
  line L1 (-29, 2) -> (-61, 2)
  line L2 (-61, 2) -> (-64, 27)
  line L3 (-64, 27) -> (-64, 13)
  line L4 (-64, 13) -> (-85, 13)
  line L5 (-85, 13) -> (-85, 0)
  line L6 (-85, 0) -> (-5, 0)
  line L7 (-5, 0) -> (-5, 13)
  line L8 (-5, 13) -> (-26, 13)
  line L9 (-26, 13) -> (-26, 27)
  line L10 (-64, 13) -> (-62.32, 13)
  line L11 (-26, 13) -> (-27.68, 13)
  constraint coincident L3.end L4.start
  constraint coincident L2 L10.end
  constraint perpendicular L3 L10
  constraint coincident L8.end L9.start
  constraint coincident L0 L11.end
  constraint perpendicular L9 L11
extrude "Extrude58" cut sketch "Sketch38" against normal blind 30 contours L0 L9 L11 | L2 L3 L10

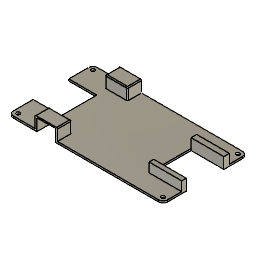
design "BASE"
Autodesk Fusion 360 part; units mm, degrees
sketch "Sketch1" plane through (0, 0, 0) normal (0, 0, 1) x (1, 0, 0)
  line L0 (0, 0) -> (165, 0)
  line L1 (165, 0) -> (165, 90)
  line L2 (165, 90) -> (0, 90)
  line L3 (0, 90) -> (0, 0)
  dimension "d1" = 165
  dimension "d2" = 90
  constraint horizontal L0
  constraint vertical L1
  constraint horizontal L2
  constraint vertical L3
  constraint coincident L0.start L3.end
  measures "d1" distance of L0.start L0.end
  measures "d2" distance of L0.start L2.end
extrude "Extrude1" add sketch "Sketch1" along normal blind 3
fillet "Fillet1" radius 5 1 edges at (0, 0, 1.5)
fillet "Fillet1" radius 5 3 edges at (0, 90, 1.5) (165, 90, 1.5) (165, 0, 1.5)